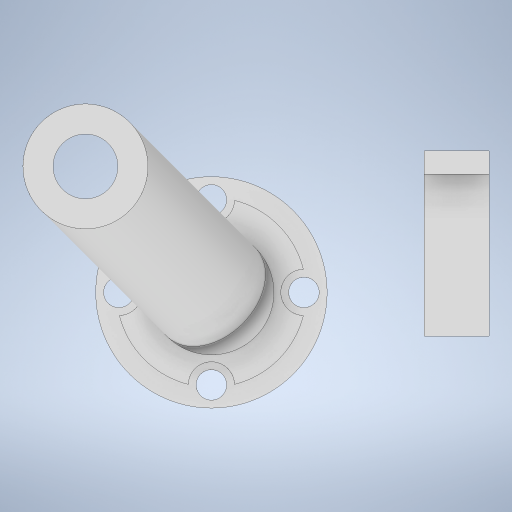
# Autodesk Inventor part: Support_RS
Saved by Autodesk Inventor 2024 (Build 280153000, 153)
## iProperties
Created: 2024-02-20
Part Number: Support_RS
Material: Genérico
Document SubType Name: Modeling
Designer: yovan
Density: 1 g/cm^3
Appearance: Valor por defecto
Author: yovan
Autodesk Inventor part; units mm, degrees
sketch "Boceto1" plane through (0, 0, 0) normal (1, 0, 0) x (0, 1, 0)
  circle A0 centre (0, 0) radius 25
  dimension "d0" = 50
  constraints: 1 centre point, 1 coincident
  measures "d0" diameter of A0
extrude "Extrusión1" add sketch "Boceto1" against normal blind 6
sketch "Boceto2" plane through (0, 0, 0) normal (1, 0, 0) x (0, 0, -1)
  circle A0 centre (0, 0) radius 20
  point P0 (20, 0)
  point P1 (0, -20)
  point P2 (-20, 0)
  point P3 (0, 20)
  dimension "d9" = 40
  constraints: 4 point on circle, 1 centre point, 1 coincident
  measures "d9" diameter of A0
hole "Agujero1" at (0, 0, -20) at (0, -20, 0) at (0, 0, 20) at (0, 20, 0) direction (-1, 0, 0) diameter 6.6 end through all clearance for "Tornillo para maquinaria de cabeza plana" size "M6" standard "Perfil M métrico ANSI"
sketch "Boceto3" plane through (0, 0, 0) normal (1, 0, 0) x (0, 0, -1)
  circle A0 centre (0, 0) radius 13.5
  dimension "d18" = 27
  constraints: 1 centre point
  measures "d18" diameter of A0
extrude "Extrusión2" add sketch "Boceto3" along normal blind 40
fillet "Empalme de cara1" radius 7 1 edges at (0, 0, 13.5)
sketch "Boceto4" plane through (0, 0, 0) normal (1, 0, 0) x (0, 0, -1)
  point P0 (0, 0)
sketch "Boceto5" plane through (0, 0, 0) normal (1, 0, 0) x (0, 0, -1)
  circle A0 centre (0, -20) radius 3.3 projected
  circle A1 centre (0, -20) radius 5
  point P0 (0, 0)
  dimension "d22" = 10
  constraints: 1 centre point, 1 coincident
  measures "d22" diameter of A1
extrude "Extrusión3" cut sketch "Boceto5" along normal blind 10
pattern_circular "Patrón circular1" count 4 over 360 about axis through (0, 0, 0) along (-1, 0, 0) of "Extrusión3"
sketch "Boceto16" plane through (40, 0, 0) normal (1, 0, 0) x (0, 0, -1)
  line L0 (9.5459, -9.5459) -> (4.773, -14.3189)
  constraints: 2 end point
ref_plane "Plano de trabajo5" through (40, -9.5459, -9.5459) normal (0.7071068, 0.5, 0.5) x (0, -0.7071068, 0.7071068)
split "Dividir2" plane through (40, -9.5459, -9.5459) removes the side toward (0.7071068, 0.5, 0.5)
sketch "Boceto18" plane through (-6, 0, 0) normal (-1, 0, 0) x (0, 0, 1)
  line L0 (0, 0) -> (17.6777, 17.6777)
  circle A0 centre (0, 0) radius 25 projected
  line L1 (0, 0) -> (25, 0) construction
  line L2 (17.6777, 17.6777) -> (25.9377, 9.4176)
  dimension "d57" = 45
  constraints: 6 end point, 1 equal length, 1 horizontal, 1 perpendicular, 2 other
  measures "d57" angle of L1 L0
ref_plane "Plano de trabajo6" through (-6, 17.6777, 17.6777) normal (0, 0.7071068, 0.7071068) x (0, -0.7071068, 0.7071068)
sketch "Boceto19" plane through (0, 0, 0) normal (1, 0, 0) x (0, 0, -1)
  circle A0 centre (0, 0) radius 25 projected
  line L0 (0, 0) -> (-27.2236, 27.2236)
  line L1 (0, 0) -> (38.5, 0) construction
  dimension "d59" = 38.5
  dimension "d60" = 135
  constraints: 4 end point, 1 equal length, 1 horizontal
  measures "d59" distance of L0.start L0.end
  measures "d60" angle of L1 L0
sketch "Boceto20" plane through (-6, 17.6777, 17.6777) normal (0, 0.7071068, 0.7071068) x (0, -0.7071068, 0.7071068)
  line L0 (0, 6) -> (0, 19)
  line L1 (0, 19) -> (10.4186, 19)
  constraints: 4 end point, 1 horizontal, 1 vertical
ref_plane "Plano de trabajo7" through (13, 17.6777, 17.6777) normal (1, 0, 0) x (0, -0.7071068, 0.7071068)
sketch "Boceto21" plane through (13, 17.6777, 17.6777) normal (1, 0, 0) x (0, -0.7071068, 0.7071068)
  circle A0 centre (0, 25) radius 25 projected
  line L0 (0, 0) -> (0, -13.5)
  circle A1 centre (0, -13.5) radius 13.5
  circle A2 centre (0, -13.5) radius 9
  dimension "d64" = 13.5
  dimension "d65" = 18
  constraints: 2 coincident, 2 end point, 2 vertical alignment, 1 centre point, 1 vertical, 3 other
  measures "d64" distance of L0.start L0.end
  measures "d65" diameter of A2
extrude "Extrusión6" add sketch "Boceto21" along normal blind 132 contours A1
sketch "Boceto22" plane through (26.5, 0, 0) normal (0.7071068, 0.5, 0.5) x (0.7071068, -0.5, -0.5)
  circle A0 centre (0, 0) radius 13.5
  point P0 (-18.7383, 0)
  dimension "d68" = 27
  constraints: 1 centre point
  measures "d68" diameter of A0
extrude "Extrusión7" add sketch "Boceto22" along normal up to next
sketch "Boceto23" plane through (145, 27.2236, 27.2236) normal (1, 0, 0) x (0, 0, -1)
  circle A0 centre (0, 0) radius 13.5
  circle A1 centre (0, 0) radius 7
  point P0 (27.2236, -27.2236)
  dimension "d71" = 27
  dimension "d72" = 14
  constraints: 2 centre point, 1 coincident
  measures "d71" diameter of A0
  measures "d72" diameter of A1
extrude "Extrusión8" add sketch "Boceto23" along normal blind 7
sketch "Boceto24" plane through (13, 17.6777, 17.6777) normal (1, 0, 0) x (0, -0.7071068, 0.7071068)
  circle A0 centre (0, -13.5) radius 13.5 projected
  line L0 (0, -27) -> (11.147, -27)
  point P0 (0, 25)
  constraints: 2 end point, 2 horizontal, 1 vertical alignment, 1 other
ref_plane "Plano de trabajo8" through (13, 36.7696, 36.7696) normal (0, -0.7071068, -0.7071068) x (0, -0.7071068, 0.7071068)
sketch "Boceto25" plane through (13, 36.7696, 36.7696) normal (0, -0.7071068, -0.7071068) x (0, -0.7071068, 0.7071068)
  line L0 (-13.5, 0) -> (13.5, 0) projected
  line L1 (0, 0) -> (0, -5)
  line L2 (0, -5) -> (-7, -5)
  line L3 (-7, -5) -> (7, -5)
  line L4 (7, -5) -> (7, -10)
  line L5 (7, -10) -> (-7, -10)
  line L6 (-7, -10) -> (-7, -5)
  dimension "d76" = 5
  dimension "d77" = 7
  dimension "d78" = 14
  dimension "d79" = 5
  constraints: 12 end point, 2 horizontal, 2 parallel, 1 midpoint, 1 perpendicular, 1 vertical
  measures "d76" distance of L1.start L1.end
  measures "d77" distance of L1.end L2.end
  measures "d78" distance of L4.end L5.end
  measures "d79" distance of L3.end L4.end
extrude "Extrusión9" cut sketch "Boceto25" along normal blind 27
sketch "Boceto27" plane through (-6, 0, 0) normal (-1, 0, 0) x (0, 0, 1)
  line L0 (-46.002, 30.5636) -> (-60.002, 30.5636)
  line L1 (-60.002, 30.5636) -> (-60.002, -9.4364)
  line L2 (-60.002, -9.4364) -> (-46.002, -9.4364)
  line L3 (-46.002, -9.4364) -> (-46.002, 30.5636)
  point P0 (0, 0)
  dimension "d83" = 14
  dimension "d84" = 40
  constraints: 8 end point, 2 parallel, 1 horizontal, 1 perpendicular
  measures "d83" distance of L2.end L1.end
  measures "d84" distance of L1.end L0.end
extrude "Extrusión10" add sketch "Boceto27" against normal blind 5
sketch "Boceto29" plane through (-1, 0, 0) normal (1, 0, 0) x (0, 0, -1)
  line L0 (60.002, -9.4364) -> (60.002, 30.5636) projected
  line L1 (60.002, 30.5636) -> (46.002, 30.5636)
  line L2 (46.002, 30.5636) -> (46.002, 25.5636)
  line L3 (46.002, 25.5636) -> (60.002, 25.5636)
  line L4 (60.002, 25.5636) -> (60.002, 30.5636)
  point P0 (0, 0)
  dimension "d87" = 14
  dimension "d88" = 5
  constraints: 8 end point, 2 parallel, 1 horizontal, 1 perpendicular
  measures "d87" distance of L3.end L2.end
  measures "d88" distance of L2.end L1.end
extrude "Extrusión11" add sketch "Boceto29" along normal blind 5
